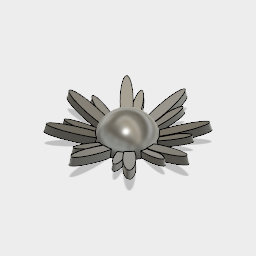
花瓣 (Autodesk Fusion 360 design; units mm, degrees)
Autodesk Fusion 360 part; units mm, degrees
sketch "草图1" plane through (0, 0, 0) normal (0, 1, 0) x (1, 0, 0)
  ellipse E0 centre (0, 0) end of major axis (6, 0) minor radius 2
  line L0 (-6, 0) -> (6, 0)
  line L1 (0, -2) -> (0, 2)
sketch "草图2" plane through (0, 0, 0) normal (0, 1, 0) x (1, 0, 0)
  ellipse E0 centre (0, 0) end of major axis (-10, 0) minor radius 2
  line L0 (10, 0) -> (-10, 0)
  line L1 (0, 2) -> (0, -2)
extrude "拉伸2" add sketch "草图2" along normal blind 3 makes body 1
move_body "移动1" bodies 1 to x (0.965926, 0, -0.258819) y (0, 1, 0) z (0.258819, 0, 0.965926) at (0.1769, 0, -2.6563)
box "长方体基本要素1" add length 3 width 3 height 3 placed x (0, 0, -1) y (-1, 0, 0) z (0, 1, 0) at (-12, 0, 0) separate body makes body 2
move_body "移动2" bodies 2 to x (1, 0, 0) y (0, 1, 0) z (0, 0, 1) at (0.8173, 0, 1.7859)
move_body "移动3" bodies 2 to x (1, 0, 0) y (0, 1, 0) z (0, 0, 1) at (-1.9419, 0, -1.6406)
move_body "移动4" bodies 1 to x (0.965926, 0, 0.258819) y (0, 1, 0) z (-0.258819, 0, 0.965926) at (-1.847, 0, 2.2572)
move_body "移动5" bodies 1 to x (0.965926, 0.258819, 0) y (-0.258819, 0.965926, 0) z (0, 0, 1) at (-0.3744, 2.8441, 0)
move_body "移动6" bodies 2 to x (1, 0, 0) y (0, 1, 0) z (0, 0, 1) at (-4.0288, 0.0995, 0)
pattern_circular "C-阵列1" count 8 over 360 about axis through (-17.1535, 3.0995, 0.1453) along (0, -1, 0) of bodies 1 makes body 3 at (-6.9548, 1.9432, 8.921) makes body 4 at (-16.1472, 1.9432, 13.5622) makes body 5 at (-25.9291, 1.9432, 10.344) makes body 6 at (-30.5704, 1.9432, 1.1515) makes body 7 at (-27.3522, 1.9432, -8.6304) makes body 8 at (-18.1597, 1.9432, -13.2716) makes body 9 at (-8.3778, 1.9432, -10.0534)
copy_body "复制和粘贴实体1" bodies 1 7 3 8 4 6 9 5 makes body 10 makes body 11 makes body 12 makes body 13 makes body 14 makes body 15 makes body 16 makes body 17
scale "缩放1" factor 0.8 about (-17.1535, 0.0995, 0.1453) bodies 10 11 12 13 14 15 16 17
move_body "移动7" bodies 11 12 16 10 13 14 17 15 to x (0.97437, 0, 0.224951) y (0, 1, 0) z (-0.224951, 0, 0.97437) at (-0.407, 0, 3.8624)
sphere "球体基本要素1" add diameter 20 placed x (1, 0, 0) y (0, 0, -1) z (0, 1, 0) at (0, 0, 0) separate body makes body 18
move_body "MoveFace1" bodies 18 to x (1, 0, 0) y (0, 1, 0) z (0, 0, 1) at (-17.6974, 1.4314, -0.1499) on bodies 18
combine "合并1" operation add target body 16 tool bodies 1 12 15 5 4 11 10 14 17 13 3 7 8 9 6 18
box "长方体基本要素2" add length 40 width 155 height 5 placed x (0, 0, 1) y (1, 0, 0) z (0, 1, 0) at (-140, 0, 0) separate body makes body 19
move_face "偏移面1" offset 30 1 faces at (-36.6667, 0, 13.3333) on bodies 19
move_body "移动8" bodies 19 to x (1, 0, 0) y (0, 1, 0) z (0, 0, 1) at (9.604, -4.0967, 0)
move_body "移动9" bodies 19 to x (1, 0, 0) y (0, 1, 0) z (0, 0, 1) at (4.847, 0, -22.4008)
combine "合并2" operation cut target body 16 tool bodies 19
hidden bodies 2
